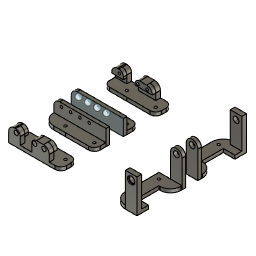
motor_mount_2 v3 (Autodesk Fusion 360 design; units mm, degrees)
Autodesk Fusion 360 part; units mm, degrees
sketch "Sketch1" plane through (0, 0, 0) normal (0, 0, 1) x (1, 0, 0) in component "motor_mount_2"
  line L0 (54.9999, 43.2813) -> (65, 43.2813)
  circle A0 centre (50, 13.2813) radius 1.125
  line L1 (55, 47.2813) -> (65, 47.2813)
  arc A1 (55, 47.2813) -> (45, 37.2813) centre (55, 37.2813) ccw
  line L2 (45, 37.2813) -> (45, 18.2813)
  circle A2 centre (50, 38.2813) radius 1.125
  line L3 (-35, 48) -> (-34.9999, 48)
  line L4 (-45, 48) -> (-35, 48)
  line L5 (-10, 34) -> (-25, 34)
  circle A3 centre (-30, 14) radius 1.125
  line L6 (-34.9999, 48) -> (-25, 48)
  line L7 (-10, 19) -> (-25, 19)
  line L8 (-10.0001, 44) -> (-10.0001, 48)
  line L9 (-25, 44) -> (-10.0001, 44)
  circle A4 centre (-30, 39) radius 1.125
  line L10 (-45, 48) -> (-45, 41)
  line L11 (-25, 48) -> (-10.0001, 48)
  line L12 (-10.0001, 48) -> (-10, 48)
  line L13 (-35, 44) -> (-45, 44)
  line L14 (-25, 44) -> (-25, 48)
  circle A5 centre (-5, 39) radius 1.125
  circle A6 centre (-5, 14) radius 1.125
  line L15 (54.9999, 43.2813) -> (55, 47.2813)
  line L16 (-35, 44) -> (-35, 48)
  line L17 (-25, 34) -> (-40, 34)
  line L18 (-10, 34) -> (-5, 34)
  line L19 (-25, 19) -> (-35, 19)
  line L20 (-10, 19) -> (-5, 19)
  line L21 (0, 14) -> (0, 9)
  line L22 (45, 18.2813) -> (45, 8.2812)
  line L23 (0, 9) -> (-45, 8.9999)
  line L24 (0, 9) -> (0, 6)
  line L25 (-45, 8.9999) -> (-45, 6)
  line L26 (-45, 6) -> (0, 6)
  line L27 (45, 8.2812) -> (45, 5.2812)
  line L28 (55, 37.2813) -> (65, 37.2813)
  line L29 (55, 37.2813) -> (55, 8.2812)
  line L30 (55, 8.2812) -> (55, 5.2812)
  line L31 (45, 8.2812) -> (55, 8.2812)
  line L32 (45, 5.2812) -> (55, 5.2812)
  line L33 (65, 43.2813) -> (65, 37.2813)
  line L34 (65, 47.2813) -> (65, 43.2813)
  line L35 (-45, 41) -> (-45, 39)
  line L36 (-45, 9) -> (-45, 8.9999)
  arc A7 (-35, 19) -> (-45, 9) centre (-35, 9) ccw
  arc A8 (0, 14) -> (-5, 19) centre (-5, 14) ccw
  arc A9 (-45, 39) -> (-40, 34) centre (-40, 39) ccw
  line L37 (-10, 48) -> (-5, 48)
  line L38 (0, 43) -> (0, 39)
  arc A10 (0, 43) -> (-5, 48) centre (-5, 43) ccw
  arc A11 (-5, 34) -> (0, 39) centre (-5, 39) ccw
  line L39 (55, 5.2812) -> (65, 5.2813)
  line L40 (55, 8.2812) -> (65, 8.2812)
  line L41 (65, 8.2812) -> (65, 5.2813)
  line L42 (65, 8.2812) -> (65, 9.2812)
  line L43 (56, 18.2812) -> (55, 18.2812)
  arc A12 (65, 9.2812) -> (56, 18.2812) centre (56, 9.2812) ccw
  point P0 (-30, 39)
  point P1 (65, 18.2812)
  dimension "d8" = 3
  dimension "d9" = 10
  dimension "d10" = 5
  dimension "d11" = 5
  dimension "d12" = 5
  dimension "d13" = 5
  constraint perpendicular L23 L25
  constraint perpendicular L24 L26
  constraint coincident A1.centre L28.start
  constraint perpendicular L29 L31
  constraint perpendicular L0 L33
  constraint perpendicular L0 L34
  constraint perpendicular L17 L35
  constraint tangent L19 A7
  constraint tangent L36 A7
  constraint tangent L20 A8
  constraint tangent L21 A8
  constraint tangent L17 A9
  constraint tangent L35 A9
  constraint horizontal L37
  constraint tangent L37 A10
  constraint tangent L38 A10
  constraint tangent L38 A11
  constraint tangent L18 A11
  constraint perpendicular L30 L39
  constraint perpendicular L29 L40
  constraint perpendicular L39 L41
  constraint perpendicular L40 L42
  constraint coincident L29 L43.end
  constraint perpendicular L29 L43
  constraint coincident P1 L43
  constraint coincident P1 L42
  constraint tangent L43 A12
  constraint tangent L42 A12
  measures "d8" distance of L22.end L27.end
  measures "d9" radius of A7
  measures "d10" radius of A8
  measures "d11" radius of A9
  measures "d12" radius of A10
  measures "d13" radius of A11
extrude "Extrude1" add sketch "Sketch1" along normal blind 3 contours L0 A1 L2 L15 L22 L28 L29 L31 L33 | L29 L40 L42 L43 A12 | L5 L6 L8 L9 L10 L13 L14 L16 L17 L18 L35 A9 L37 L38 A10 A11 | L7 L19 L20 L21 L23 A7 A8 makes body 1 at (-20, 40.6667, 0) makes body 2 at (-20, 15.4456, 0) makes body 3 at (50.028, 24.574, 0) in component "motor_mount_2"
extrude "Extrude2" add sketch "Sketch1" along normal blind 13.6 contours L4 L10 L13 L16 | L8 L9 L11 L14 | L23 L24 L25 L26 bodies 1 2 in component "motor_mount_2"
sketch "Sketch2" plane through (0, 6, 0) normal (0, -1, 0) x (1, 0, 0) in component "motor_mount_2"
  line L0 (-45, 0) -> (0, 0)
  line L1 (0, 0) -> (0, 13.6)
  line L2 (0, 13.6) -> (-45, 13.6)
  line L3 (-45, 13.6) -> (-45, 0)
  line L4 (-40, 13.6) -> (-38, 13.6)
  arc A0 (-40, 13.6) -> (-45, 8.6) centre (-40, 8.6) ccw
  line L5 (-45, 6.8) -> (-45, 13.6)
  line L6 (-45, 13.6) -> (-38, 13.6)
  line L7 (-45, 13.6) -> (-38, 13.6)
  dimension "d22" = 5
  constraint coincident L2 L4.end
  constraint perpendicular L3 L4
  constraint midpoint L3 L5.start
  constraint tangent L4 A0
  constraint coincident L2.end L3.start
  constraint perpendicular L5 L6
  constraint perpendicular L3 L7
  measures "d22" radius of A0
extrude "Extrude3" cut sketch "Sketch2" against normal blind 3 contours L2 L3 A0 L5 L6 L7 bodies 2 in component "motor_mount_2"
sketch "Sketch1 (2)" plane through (0, 6, 0) normal (0, -1, 0) x (1, 0, 0)
  arc A0 (-40, 13.6) -> (-45, 8.6) centre (-40, 8.6) ccw
  line L0 (-45, 8.6) -> (-45, 0)
  line L1 (-45, 0) -> (0, 0)
  line L2 (0, 0) -> (0, 13.6)
  line L3 (0, 13.6) -> (-40, 13.6)
  circle A1 centre (-38.5, 10.5) radius 1.125
  circle A2 centre (-30.5, 10.5) radius 1.125
  circle A3 centre (-22.5, 10.5) radius 1.125
  circle A4 centre (-14.5, 10.5) radius 1.125
  dimension "d27" = 2.25
  dimension "d28" = 8
  dimension "d29" = 8
  dimension "d30" = 8
  dimension "d31" = 2.25
  dimension "d32" = 2.25
  dimension "d33" = 2.25
  measures "d27" diameter of A1
  measures "d28" distance of A1.centre A2.centre
  measures "d29" distance of A2.centre A3.centre
  measures "d30" distance of A3.centre A4.centre
  measures "d31" diameter of A2
  measures "d32" diameter of A3
  measures "d33" diameter of A4
hole "Hole1" at (-38.5, 6, 10.5) direction (0, 1, 0) diameter 2.25 depth 7 tip angle 118 bodies 2 in component "motor_mount_2"
hole "Hole2" at (-30.5, 6, 10.5) direction (0, 1, 0) diameter 2.25 depth 7 tip angle 118 bodies 2 in component "motor_mount_2"
hole "Hole3" at (-22.5, 6, 10.5) direction (0, 1, 0) diameter 2.25 depth 7 tip angle 118 bodies 2 in component "motor_mount_2"
hole "Hole4" at (-14.5, 6, 10.5) direction (0, 1, 0) diameter 2.25 depth 7 tip angle 118 bodies 2 in component "motor_mount_2"
sketch "Sketch2 (2)" plane through (0, 48, 0) normal (0, 1, 0) x (-1, 0, 0)
  line L0 (5, 0) -> (45, 0)
  line L1 (45, 0) -> (45, 13.6)
  line L2 (45, 13.6) -> (35, 13.6)
  line L3 (35, 13.6) -> (35, 3)
  line L4 (35, 3) -> (25, 3)
  line L5 (25, 3) -> (25, 13.6)
  line L6 (25, 13.6) -> (10.0001, 13.6)
  line L7 (10.0001, 13.6) -> (10.0001, 3)
  line L8 (10.0001, 3) -> (5, 3)
  line L9 (5, 3) -> (5, 0)
  circle A0 centre (38.5, 10.5) radius 1.125
  circle A1 centre (22.5, 10.5) radius 1.125
  circle A2 centre (14.5, 10.5) radius 1.125
  dimension "d48" = 2.25
  dimension "d49" = 16
  dimension "d50" = 8
  dimension "d51" = 2.25
  dimension "d52" = 2.25
  measures "d48" diameter of A0
  measures "d49" distance of A0.centre A1.centre
  measures "d50" distance of A1.centre A2.centre
  measures "d51" diameter of A1
  measures "d52" diameter of A2
hole "Hole5" at (-38.5, 48, 10.5) direction (0, -1, 0) diameter 2.25 depth 7 tip angle 118 bodies 1 in component "motor_mount_2"
hole "Hole6" at (-22.5, 48, 10.4999) direction (0, -1, 0) diameter 2.25 depth 7 tip angle 118 bodies 1 in component "motor_mount_2"
hole "Hole7" at (-14.4999, 48, 10.5) direction (0, -1, 0) diameter 2.25 depth 7 tip angle 118 bodies 1 in component "motor_mount_2"
fillet "Fillet1" radius 5 1 edges at (-10.0001, 46, 13.6) on bodies 1 in component "motor_mount_2"
fillet "Fillet2" radius 4 1 edges at (-25, 46, 13.6) on bodies 1 in component "motor_mount_2"
fillet "Fillet3" radius 4 1 edges at (-35, 46, 13.6) on bodies 1 in component "motor_mount_2"
fillet "Fillet4" radius 5 1 edges at (-45, 46, 13.6) on bodies 1 in component "motor_mount_2"
sketch "Sketch3" plane through (0, 44, 0) normal (0, -1, 0) x (1, 0, 0)
  circle A0 centre (-38.5, 10.5) radius 1.125
  arc A1 (-40, 13.6) -> (-45, 8.6) centre (-40, 8.6) ccw
  line L0 (-45, 8.6) -> (-45, 3)
  line L1 (-45, 3) -> (-35, 3)
  line L2 (-35, 3) -> (-35, 9.6)
  arc A2 (-35, 9.6) -> (-39, 13.6) centre (-39, 9.6) ccw
  line L3 (-39, 13.6) -> (-40, 13.6)
  line L4 (-45, 7.522) -> (-35, 7.522)
  constraint coincident L0 L4.start
  constraint coincident L2 L4.end
  constraint perpendicular L2 L4
extrude "Extrude4" add sketch "Sketch3" along normal blind 3 contours A1 L0 L2 A2 L3 L4 bodies 1 in component "motor_mount_2"
sketch "Sketch4" plane through (0, 44, 0) normal (0, -1, 0) x (1, 0, 0)
  circle A0 centre (-14.4999, 10.5) radius 1.125
  circle A1 centre (-22.5, 10.4999) radius 1.125
  arc A2 (-21, 13.6) -> (-25, 9.6) centre (-21, 9.6) ccw
  line L0 (-25, 9.6) -> (-25, 3)
  line L1 (-25, 3) -> (-10.0001, 3)
  line L2 (-10.0001, 3) -> (-10.0001, 8.6)
  arc A3 (-10.0001, 8.6) -> (-15.0001, 13.6) centre (-15.0001, 8.6) ccw
  line L3 (-15.0001, 13.6) -> (-21, 13.6)
  line L4 (-10.0001, 8.6) -> (-25, 8.6)
  constraint coincident L2.end A3.start
  constraint coincident L0 L4.end
  constraint perpendicular L0 L4
extrude "Extrude5" add sketch "Sketch4" along normal blind 3 contours A2 L0 A3 L3 L4 bodies 1 in component "motor_mount_2"
hole "Hole8" at (-14.4999, 48, 10.5) direction (0, -1, 0) diameter 3.7 depth 3.5 tip angle 118 bodies 1 in component "motor_mount_2"
hole "Hole9" at (-22.5, 48, 10.4999) direction (0, -1, 0) diameter 3.7 depth 3.5 tip angle 118 bodies 1 in component "motor_mount_2"
hole "Hole10" at (-38.5, 48, 10.5) direction (0, -1, 0) diameter 3.7 depth 3.5 tip angle 118 bodies 1 in component "motor_mount_2"
extrude "Extrude6" add sketch "Sketch1" along normal blind 30 contours L0 L1 L15 L34 | L30 L39 L40 L41 bodies 3 in component "motor_mount_2"
sketch "Sketch5" plane through (0, 5.2812, 0) normal (0.000001, -1, 0) x (1, 0.000001, 0)
  line L0 (55, 0) -> (65, 0)
  line L1 (65, 0) -> (65, 30)
  line L2 (65, 30) -> (55, 30)
  line L3 (55, 30) -> (55, 0)
  line L4 (60, 30) -> (60, 24)
  circle A0 centre (60, 24) radius 1.275
  dimension "d81" = 6
  dimension "d82" = 2.55
  constraint midpoint L2 L4.start
  constraint perpendicular L2 L4
  constraint coincident L4.end A0.centre
  measures "d81" distance of L4.start L4.end
  measures "d82" diameter of A0
hole "Hole11" at (60, 5.2813, 24) direction (-0.000001, 1, 0) diameter 2.55 depth 7 tip angle 118 bodies 3 in component "motor_mount_2"
extrude "Extrude7" cut 1 faces at (58.3333, 7.2812, 30) along direction (0, 0, -1) blind 3 on bodies 3 bodies 3 in component "motor_mount_2"
sketch "Sketch6" plane through (0, 47.2812, 0) normal (-0.000001, 1, 0) x (-1, -0.000001, 0)
  line L0 (-65, 0) -> (-55, 0)
  line L1 (-55, 0) -> (-55, 3)
  line L2 (-55, 3) -> (-55, 30)
  line L3 (-55, 30) -> (-65, 30)
  line L4 (-65, 30) -> (-65, 0)
hole "Hole12" at (60, 5.2813, 24) direction (-0.000001, 1, 0) diameter 2.55 depth 7 tip angle 118 counterbore diameter 3.15 counterbore depth 1 bodies 3 in component "motor_mount_2"
hole "Hole13" at (59.9999, 47.2813, 23.9997) direction (0.000001, -1, 0) diameter 5 depth 7 tip angle 118 counterbore diameter 6.3 counterbore depth 1 bodies 3 in component "motor_mount_2"
extrude "Extrude8" add 1 faces at (58.3333, 7.2812, 27) along direction (0, 0, 1) blind 3 on bodies 3 bodies 3 in component "motor_mount_2"
hole "Hole14" at (60, 5.2813, 24) direction (-0.000001, 1, 0) diameter 5 depth 7 tip angle 118 bodies 3 in component "motor_mount_2"
extrude "Extrude9" cut 1 faces at (58.3333, 7.2812, 30) along direction (0, 0, -1) blind 1.5 on bodies 3 bodies 3 in component "motor_mount_2"
fillet "Fillet5" radius 5 1 edges at (55, 6.7812, 28.5) on bodies 3 in component "motor_mount_2"
fillet "Fillet6" radius 5 1 edges at (65, 6.7813, 28.5) on bodies 3 in component "motor_mount_2"
extrude "Extrude10" cut 1 faces at (58.3333, 44.6146, 30) along direction (0, 0, -1) blind 1 on bodies 3 bodies 3 in component "motor_mount_2"
mirror "Mirror1" about plane through (0, 0, 0) normal (0, 1, 0) of bodies 3 2 1 makes body 4 at (-26.5832, -45.3656, 0) makes body 5 at (-22.5, -6, 3.125) makes body 6 at (50.028, -24.574, 0) in component "motor_mount_2"
component "motor_mount_2" placed x (1, 0, 0) y (0, 1, 0) z (0, 0, 1) at (0, 0, 0)
